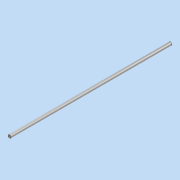
# Autodesk Inventor part: Führung
Saved by Autodesk Inventor 2021 (Build 250183000, 183)
## iProperties
Created: 2024-03-15
Part Number: Führung
Material: Generic
Document SubType Name: Modeling
Designer: Nokia
Density: 1 g/cm^3
Appearance: Stainless - Brushed
Author: Nokia
Autodesk Inventor part; units mm, degrees
ref_plane "YZ Plane" through (0, 0, 0) normal (1, 0, 0) x (0, 1, 0)
ref_plane "XZ Plane" through (0, 0, 0) normal (0, 1, 0) x (-1, 0, 0)
ref_plane "XY Plane" through (0, 0, 0) normal (0, 0, 1) x (1, 0, 0)
sketch "Sketch1" plane through (0, 0, 0) normal (0, 0, 1) x (1, 0, 0)
  circle A0 centre (0, 0) radius 13
  dimension "d0" = 26
  constraints: 1 centre point, 1 coincident
  measures "d0" diameter of A0
extrude "Extrusion1" add sketch "Sketch1" along normal blind 1350
sketch "Sketch2" plane through (0, 0, 1350) normal (0, 0, 1) x (1, 0, 0)
  line L0 (0, 0) -> (0, 6.5)
  circle A0 centre (0, 6.5) radius 3.5
  circle A1 centre (-5.6292, -3.25) radius 3.5
  circle A2 centre (5.6292, -3.25) radius 3.5
  dimension "d5" = 6.5
  dimension "d6" = 7
  dimension "d7" = 360
  constraints: 3 centre point, 2 end point, 1 coincident, 1 vertical, 7 other
  measures "d5" distance of L0.start L0.end
  measures "d6" diameter of A0
hole "Hole1" at (0, 6.5, 1350) at (5.6292, -3.25, 1350) at (-5.6292, -3.25, 1350) direction (0, 0, -1) diameter 4.134 depth 49 tip angle 118 thread size "M5x0.8" class "6H" standard "ISO Metric profile"
body "Solid1"
